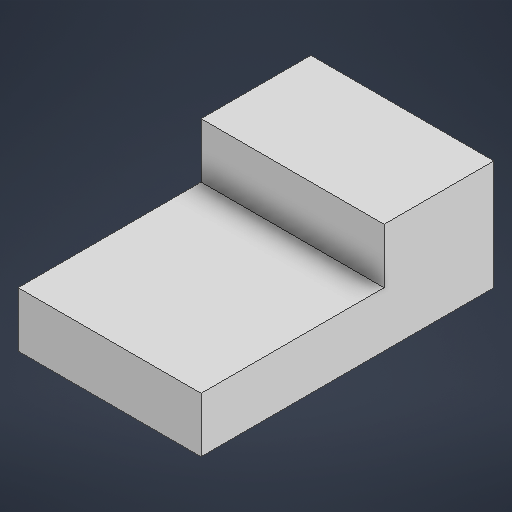
# Autodesk Inventor part: Part3
Saved by Autodesk Inventor 2026 (Build 300175050, 175E)
## iProperties
Created: 2026-03-12
Part Number: Part3
Material: Generic
Document SubType Name: Modeling
Designer: Administrator
Density: 1 g/cm^3
Appearance: Default
Author: Administrator
Autodesk Inventor part; units mm, degrees
ref_plane "YZ Plane" through (0, 0, 0) normal (1, 0, 0) x (0, 1, 0)
ref_plane "XZ Plane" through (0, 0, 0) normal (0, 1, 0) x (-1, 0, 0)
ref_plane "XY Plane" through (0, 0, 0) normal (0, 0, 1) x (1, 0, 0)
sketch "Sketch1" plane through (0, 0, 0) normal (1, 0, 0) x (0, 1, 0)
  line L0 (0, 0) -> (0, -40)
  line L1 (0, -40) -> (15, -40)
  line L2 (15, -40) -> (15, -25)
  line L3 (15, -25) -> (7.5, -25)
  line L4 (7.5, -25) -> (7.5, 0)
  line L5 (7.5, 0) -> (0, 0)
  dimension "d0" = 15
  dimension "d1" = 7.5
  dimension "d2" = 15
  dimension "d3" = 40
  constraints: 12 end point, 4 perpendicular, 1 horizontal, 1 vertical
  measures "d0" distance of L0.end L1.end
  measures "d1" distance of L4.end L0.start
  measures "d2" distance of L1.end L2.end
  measures "d3" distance of L0.start L0.end
extrude "Extrusion1" add sketch "Sketch1" against normal blind 25
body "Solid1"
